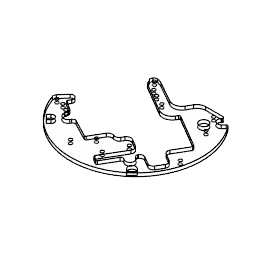
ElectronicsPlate_v18 (Autodesk Fusion 360 design; units mm, degrees)
Autodesk Fusion 360 part; units mm, degrees
sketch "Sketch1" plane through (0, 0, 0) normal (0, 0, 1) x (1, 0, 0)
  line L0 (24.0462, -23.2611) -> (4.7349, -11.9168)
  line L1 (4.7349, -11.9168) -> (-10, -37)
  line L2 (-37, -23) -> (-46.9743, -17.1407)
  line L3 (-46.9743, -17.1407) -> (-43.6068, -11.1794)
  line L4 (-43.6068, -11.1794) -> (-48.5198, -8.4041)
  circle A0 centre (0, 0) radius 60.0314
  line L5 (-48.5198, -8.4041) -> (-57.1777, -18.2887)
  line L6 (24.0462, -23.2611) -> (9.3113, -48.3442)
  line L7 (9.3113, -48.3442) -> (14.5577, -51.4261)
  line L8 (14.5577, -51.4261) -> (30.7123, -23.9261)
  line L9 (30.7123, -23.9261) -> (43.6758, -31.5414)
  line L10 (43.6758, -31.5414) -> (50.8465, -19.3347)
  line L11 (50.8465, -19.3347) -> (38.1044, -11.8495)
  line L12 (38.1044, -11.8495) -> (48.0926, 5.1535)
  line L13 (48.0926, 5.1535) -> (17.0156, 23.4093)
  line L14 (17.0156, 23.4093) -> (11.0792, 13.3037)
  line L15 (11.0792, 13.3037) -> (-19.6069, 31.3299)
  line L16 (-19.6069, 31.3299) -> (-23.3154, 25.0171)
  line L17 (-23.3154, 25.0171) -> (-29.9322, 28.904)
  line L18 (-29.9322, 28.904) -> (-25, 42)
  line L19 (-25, 42) -> (-19, 42)
  line L20 (-19, 42) -> (42.8925, 42)
  line L21 (10.662, -15.3987) -> (5.2376, -24.6327)
  line L22 (5.2376, -24.6327) -> (-0.6896, -21.1508)
  line L23 (-10, -37) -> (-37, -23)
  circle A1 centre (-45.771, -21.2236) radius 1.5
  circle A2 centre (-39.7105, -24.6734) radius 1.5
  circle A3 centre (-15.397, 31.6594) radius 1.5
  circle A4 centre (-9.3343, 28.1196) radius 1.5
  circle A5 centre (-21.7816, 38.5791) radius 1.5
  circle A6 centre (33.5, 37.5) radius 1.5
  circle A7 centre (10, -41) radius 1.5
  circle A8 centre (-3.1602, -33.1428) radius 1.5
  circle A9 centre (17.5729, -23.737) radius 1.5
  line L24 (-20.4528, 42) -> (8, 26)
  line L25 (8, 26) -> (16.9974, 42)
  circle A10 centre (-14, -46) radius 1.5
  circle A11 centre (-52.5, -20) radius 1.5
  circle A12 centre (52.7114, -12.238) radius 1.5
  circle A13 centre (41, 23) radius 1.5
  circle A14 centre (34, 28) radius 4
  circle A15 centre (28.5889, -34.0006) radius 4
  circle A16 centre (-33.8774, -28.5072) radius 4
  circle A17 centre (-27.9023, 34.2937) radius 4
  circle A18 centre (-0.4273, 23.9816) radius 1.5
  line L26 (-30.3297, -30.3548) -> (-28.4208, -27.4485)
  line L27 (-37.7611, -27.5497) -> (-37, -23)
  line L28 (-19.6069, 31.3299) -> (-23.9252, 33.8667)
  dimension "d1" = 3
  dimension "d2" = 3
  dimension "d3" = 3
  dimension "d4" = 3
  dimension "d5" = 3
  dimension "d6" = 3
  dimension "d9" = 3
  dimension "d10" = 3
  dimension "d15" = 3
  dimension "d38" = 3
  dimension "d39" = 3
  dimension "d41" = 3
  dimension "d42" = 3
  dimension "d43" = 8
  dimension "d44" = 8
  dimension "d45" = 8
  dimension "d46" = 8
  dimension "d47" = 3
  constraint perpendicular L0 L1
  constraint perpendicular L1 L2
  constraint perpendicular L3 L4
  constraint coincident A0.centre origin
  constraint coincident A0 L5.end
  constraint perpendicular L0 L6
  constraint perpendicular L6 L7
  constraint perpendicular L7 L8
  constraint perpendicular L8 L9
  constraint perpendicular L9 L10
  constraint perpendicular L8 L11
  constraint perpendicular L11 L12
  constraint perpendicular L12 L13
  constraint perpendicular L13 L14
  constraint perpendicular L14 L15
  constraint perpendicular L15 L16
  constraint perpendicular L16 L17
  constraint horizontal L19
  constraint coincident A0 L20.end
  constraint parallel L19 L20
  constraint coincident L0 L21.start
  constraint perpendicular L0 L21
  constraint coincident L1 L22.end
  constraint perpendicular L1 L22
  constraint coincident L20 L24.start
  constraint coincident L20 L25.end
  constraint perpendicular L24 L25
  constraint coincident L18 A17.centre
  constraint coincident A16 L26.start
  constraint coincident L23 L26.end
  constraint coincident A16 L27.start
  constraint coincident A17 L28.end
  constraint perpendicular L16 L28
  measures "d1" diameter of A1
  measures "d2" diameter of A2
  measures "d3" diameter of A3
  measures "d4" diameter of A4
  measures "d5" diameter of A5
  measures "d6" diameter of A6
  measures "d9" diameter of A7
  measures "d10" diameter of A8
  measures "d15" diameter of A9
  measures "d38" diameter of A10
  measures "d39" diameter of A11
  measures "d41" diameter of A12
  measures "d42" diameter of A13
  measures "d43" diameter of A14
  measures "d44" diameter of A15
  measures "d45" diameter of A16
  measures "d46" diameter of A17
  measures "d47" diameter of A18
extrude "Extrude1" add sketch "Sketch1" along normal blind 3 contours L0 L1 L2 L3 L4 A0 L5 L6 L7 L8 L9 L10 L11 L12 L13 L14 L15 L18 L19 L20 L21 L22 L23 L24 L25 A15 A16 A17 L26 L27 L28
fillet "Fillet1" radius 4 4 edges at (24.0462, -23.2611, 1.5) (10.662, -15.3987, 1.5) (5.2376, -24.6327, 1.5) (-0.6896, -21.1508, 1.5)
fillet "Fillet2" radius 1 3 edges at (14.5577, -51.4261, 1.5) (9.3113, -48.3442, 1.5) (-10, -37, 1.5)
fillet "Fillet3" radius 1 1 edges at (-46.9743, -17.1407, 1.5)
fillet "Fillet4" radius 3 3 edges at (-57.1777, -18.2887, 1.5) (-48.5198, -8.4041, 1.5) (-43.6068, -11.1794, 1.5)
fillet "Fillet5" radius 3.5 4 edges at (43.6758, -31.5414, 1.5) (30.7123, -23.9261, 1.5) (38.1044, -11.8495, 1.5) (50.8465, -19.3347, 1.5)
fillet "Fillet6" radius 1 2 edges at (48.0926, 5.1535, 1.5) (17.0156, 23.4093, 1.5)
fillet "Fillet7" radius 4 2 edges at (42.8925, 42, 1.5) (-25, 42, 1.5)
fillet "Fillet8" radius 8.5 1 edges at (11.0792, 13.3037, 1.5)
fillet "Fillet9" radius 8 2 edges at (16.9974, 42, 1.5) (8, 26, 1.5)
fillet "Fillet10" radius 14.5 1 edges at (-20.4528, 42, 1.5)
fillet "Fillet11" radius 2.5 2 edges at (-28.4208, -27.4485, 1.5) (-37, -23, 1.5)
fillet "Fillet12" radius 2 2 edges at (24.6023, -34.3272, 1.5) (26.9331, -30.3594, 1.5)
fillet "Fillet13" radius 2.5 2 edges at (-23.9252, 33.8667, 1.5) (-26.4925, 38.037, 1.5)
sketch "Sketch4" plane through (0, 0, 3) normal (0, 0, 1) x (-1, 0, 0)
  arc A0 (25.2969, -40.5706) -> (25.1203, -37.1677) centre (23.3814, -38.964) ccw
  arc A1 (23.9538, -34.9334) -> (25.1203, -37.1677) centre (27.9023, -34.2937) ccw
  arc A2 (23.9538, -34.9334) -> (22.7523, -33.1776) centre (21.486, -35.3332) ccw
  line L0 (22.7523, -33.1776) -> (-3.7502, -17.609)
  arc A3 (-3.7502, -17.609) -> (-15.3845, -20.6327) centre (-8.0555, -24.938) ccw
  line L1 (-15.3845, -20.6327) -> (-16.5091, -22.5471)
  arc A4 (-17.8778, -22.9028) -> (-16.5091, -22.5471) centre (-17.3713, -22.0406) ccw
  line L2 (-17.8778, -22.9028) -> (-47.2303, -5.66)
  arc A5 (-47.5861, -4.2912) -> (-47.2303, -5.66) centre (-46.7238, -4.7977) ccw
  line L3 (-47.5861, -4.2912) -> (-39.8772, 8.8317)
  arc A6 (-39.8772, 8.8317) -> (-41.1222, 13.6223) centre (-42.895, 10.6044) ccw
  line L4 (-41.1222, 13.6223) -> (-47.8287, 17.5619)
  arc A7 (-49.0737, 22.3525) -> (-47.8287, 17.5619) centre (-46.0559, 20.5797) ccw
  line L5 (-49.0737, 22.3525) -> (-45.4486, 28.5236)
  arc A8 (-40.658, 29.7686) -> (-45.4486, 28.5236) centre (-42.4307, 26.7508) ccw
  line L6 (-40.658, 29.7686) -> (-33.7301, 25.6989)
  arc A9 (-33.7301, 25.6989) -> (-28.9395, 26.9439) centre (-31.9573, 28.7167) ccw
  line L7 (-28.9395, 26.9439) -> (-28.7377, 27.2875)
  arc A10 (-28.7377, 27.2875) -> (-29.8377, 30.2005) centre (-30.4621, 28.3005) ccw
  arc A11 (-25.8777, 36.9416) -> (-29.8377, 30.2005) centre (-28.5889, 34.0006) ccw
  arc A12 (-25.8777, 36.9416) -> (-22.7977, 37.3991) centre (-24.5222, 38.4121) ccw
  line L8 (-22.7977, 37.3991) -> (-15.0642, 50.5639)
  arc A13 (-13.6954, 50.9196) -> (-15.0642, 50.5639) centre (-14.2019, 50.0574) ccw
  line L9 (-13.6954, 50.9196) -> (-10.1735, 48.8507)
  arc A14 (-9.8178, 47.482) -> (-10.1735, 48.8507) centre (-10.6801, 47.9885) ccw
  line L10 (-9.8178, 47.482) -> (-22.0201, 26.71)
  arc A15 (-22.0201, 26.71) -> (-20.5972, 21.235) centre (-18.5712, 24.6839) ccw
  line L11 (-20.5972, 21.235) -> (-14.1109, 17.4247)
  arc A16 (-14.1109, 17.4247) -> (-8.636, 18.8476) centre (-12.0849, 20.8736) ccw
  line L12 (-8.636, 18.8476) -> (-7.2636, 21.1837)
  arc A17 (-2.2942, 22.8574) -> (-7.2636, 21.1837) centre (-3.8147, 19.1577) ccw
  arc A18 (-2.2942, 22.8574) -> (2.6753, 24.5311) centre (-0.7737, 26.5572) ccw
  line L13 (2.6753, 24.5311) -> (9.5195, 36.1821)
  arc A19 (10.8421, 36.5634) -> (9.5195, 36.1821) centre (10.3818, 35.6756) ccw
  line L14 (10.8421, 36.5634) -> (26.4186, 28.4867)
  arc A20 (26.4186, 28.4867) -> (29.659, 29.3336) centre (27.5694, 30.706) ccw
  line L15 (29.659, 29.3336) -> (30.3297, 30.3548)
  arc A21 (37.7611, 27.5497) -> (30.3297, 30.3548) centre (33.8774, 28.5072) ccw
  line L16 (37.7611, 27.5497) -> (37.2839, 24.6967)
  arc A22 (37.2839, 24.6967) -> (38.4833, 22.1286) centre (39.7496, 24.2842) ccw
  line L17 (38.4833, 22.1286) -> (46.1265, 17.6387)
  arc A23 (46.4907, 16.2846) -> (46.1265, 17.6387) centre (45.62, 16.7765) ccw
  line L18 (46.4907, 16.2846) -> (45.0823, 13.7915)
  arc A24 (45.0823, 13.7915) -> (46.2188, 9.7039) centre (47.6944, 12.3159) ccw
  line L19 (46.2188, 9.7039) -> (46.3953, 9.6042)
  arc A25 (46.3953, 9.6042) -> (50.1275, 10.2396) centre (47.8708, 12.2163) ccw
  line L20 (50.1275, 10.2396) -> (56.0414, 16.9914)
  arc A26 (56.0414, 16.9914) -> (56.6139, 19.9658) centre (53.7847, 18.968) ccw
  arc A27 (56.6139, 19.9658) -> (-44.1162, -40.7128) centre (0, 0) ccw
  arc A28 (-44.1162, -40.7128) -> (-41.1766, -42) centre (-41.1766, -38) ccw
  line L21 (-41.1766, -42) -> (-21.6768, -42)
  arc A29 (-21.6768, -42) -> (-14.7037, -37.9212) centre (-21.6768, -34) ccw
  line L22 (-14.7037, -37.9212) -> (-11.9212, -32.9731)
  arc A30 (-1.0269, -29.9212) -> (-11.9212, -32.9731) centre (-4.9481, -36.8943) ccw
  line L23 (-1.0269, -29.9212) -> (17.4875, -40.3325)
  arc A31 (17.4875, -40.3325) -> (22.2322, -42) centre (24.5947, -27.6938) ccw
  arc A32 (22.2322, -42) -> (25.2969, -40.5706) centre (22.2322, -38) ccw
  circle A33 centre (45.771, 21.2236) radius 1.5
  circle A34 centre (39.7105, 24.6734) radius 1.5
  circle A35 centre (15.397, -31.6594) radius 1.5
  circle A36 centre (9.3343, -28.1196) radius 1.5
  circle A37 centre (21.7816, -38.5791) radius 1.5
  circle A38 centre (-33.5, -37.5) radius 1.5
  circle A39 centre (-10, 41) radius 1.5
  circle A40 centre (3.1602, 33.1428) radius 1.5
  circle A41 centre (-17.5729, 23.737) radius 1.5
  circle A42 centre (14, 46) radius 1.5
  circle A43 centre (52.5, 20) radius 1.5
  circle A44 centre (-52.7114, 12.238) radius 1.5
  circle A45 centre (-41, -23) radius 1.5
  circle A46 centre (-34, -28) radius 4
  circle A47 centre (0.4273, -23.9816) radius 1.5
sketch "Sketch5" plane through (0, 0, 0) normal (0, 0, -1) x (1, 0, 0)
  circle A0 centre (-0.4273, -23.9816) radius 1.5
  circle A1 centre (34, -28) radius 4
  circle A2 centre (41, -23) radius 1.5
  circle A3 centre (52.7114, 12.238) radius 1.5
  circle A4 centre (-52.5, 20) radius 1.5
  circle A5 centre (-14, 46) radius 1.5
  circle A6 centre (17.5729, 23.737) radius 1.5
  circle A7 centre (-3.1602, 33.1428) radius 1.5
  circle A8 centre (10, 41) radius 1.5
  circle A9 centre (33.5, -37.5) radius 1.5
  circle A10 centre (-21.7816, -38.5791) radius 1.5
  circle A11 centre (-9.3343, -28.1196) radius 1.5
  circle A12 centre (-15.397, -31.6594) radius 1.5
  circle A13 centre (-39.7105, 24.6734) radius 1.5
  circle A14 centre (-45.771, 21.2236) radius 1.5
  arc A15 (-25.1203, -37.1677) -> (-25.2969, -40.5706) centre (-23.3814, -38.964) ccw
  arc A16 (-25.2969, -40.5706) -> (-22.2322, -42) centre (-22.2322, -38) ccw
  arc A17 (-22.2322, -42) -> (-17.4875, -40.3325) centre (-24.5947, -27.6938) ccw
  line L0 (-17.4875, -40.3325) -> (1.0269, -29.9212)
  arc A18 (11.9212, -32.9731) -> (1.0269, -29.9212) centre (4.9481, -36.8943) ccw
  line L1 (11.9212, -32.9731) -> (14.7037, -37.9212)
  arc A19 (14.7037, -37.9212) -> (21.6768, -42) centre (21.6768, -34) ccw
  line L2 (21.6768, -42) -> (41.1766, -42)
  arc A20 (41.1766, -42) -> (44.1162, -40.7128) centre (41.1766, -38) ccw
  arc A21 (44.1162, -40.7128) -> (-56.6139, 19.9658) centre (0, 0) ccw
  arc A22 (-56.6139, 19.9658) -> (-56.0414, 16.9914) centre (-53.7847, 18.968) ccw
  line L3 (-56.0414, 16.9914) -> (-50.1275, 10.2396)
  arc A23 (-50.1275, 10.2396) -> (-46.3953, 9.6042) centre (-47.8708, 12.2163) ccw
  line L4 (-46.3953, 9.6042) -> (-46.2188, 9.7039)
  arc A24 (-46.2188, 9.7039) -> (-45.0823, 13.7915) centre (-47.6944, 12.3159) ccw
  line L5 (-45.0823, 13.7915) -> (-46.4907, 16.2846)
  arc A25 (-46.1265, 17.6387) -> (-46.4907, 16.2846) centre (-45.62, 16.7765) ccw
  line L6 (-46.1265, 17.6387) -> (-38.4833, 22.1286)
  arc A26 (-38.4833, 22.1286) -> (-37.2839, 24.6967) centre (-39.7496, 24.2842) ccw
  line L7 (-37.2839, 24.6967) -> (-37.7611, 27.5497)
  arc A27 (-30.3297, 30.3548) -> (-37.7611, 27.5497) centre (-33.8774, 28.5072) ccw
  line L8 (-30.3297, 30.3548) -> (-29.659, 29.3336)
  arc A28 (-29.659, 29.3336) -> (-26.4186, 28.4867) centre (-27.5694, 30.706) ccw
  line L9 (-26.4186, 28.4867) -> (-10.8421, 36.5634)
  arc A29 (-9.5195, 36.1821) -> (-10.8421, 36.5634) centre (-10.3818, 35.6756) ccw
  line L10 (-9.5195, 36.1821) -> (-2.6753, 24.5311)
  arc A30 (-2.6753, 24.5311) -> (2.2942, 22.8574) centre (0.7737, 26.5572) ccw
  arc A31 (7.2636, 21.1837) -> (2.2942, 22.8574) centre (3.8147, 19.1577) ccw
  line L11 (7.2636, 21.1837) -> (8.636, 18.8476)
  arc A32 (8.636, 18.8476) -> (14.1109, 17.4247) centre (12.0849, 20.8736) ccw
  line L12 (14.1109, 17.4247) -> (20.5972, 21.235)
  arc A33 (20.5972, 21.235) -> (22.0201, 26.71) centre (18.5712, 24.6839) ccw
  line L13 (22.0201, 26.71) -> (9.8178, 47.482)
  arc A34 (10.1735, 48.8507) -> (9.8178, 47.482) centre (10.6801, 47.9885) ccw
  line L14 (10.1735, 48.8507) -> (13.6954, 50.9196)
  arc A35 (15.0642, 50.5639) -> (13.6954, 50.9196) centre (14.2019, 50.0574) ccw
  line L15 (15.0642, 50.5639) -> (22.7977, 37.3991)
  arc A36 (22.7977, 37.3991) -> (25.8777, 36.9416) centre (24.5222, 38.4121) ccw
  arc A37 (29.8377, 30.2005) -> (25.8777, 36.9416) centre (28.5889, 34.0006) ccw
  arc A38 (29.8377, 30.2005) -> (28.7377, 27.2875) centre (30.4621, 28.3005) ccw
  line L16 (28.7377, 27.2875) -> (28.9395, 26.9439)
  arc A39 (28.9395, 26.9439) -> (33.7301, 25.6989) centre (31.9573, 28.7167) ccw
  line L17 (33.7301, 25.6989) -> (40.658, 29.7686)
  arc A40 (45.4486, 28.5236) -> (40.658, 29.7686) centre (42.4307, 26.7508) ccw
  line L18 (45.4486, 28.5236) -> (49.0737, 22.3525)
  arc A41 (47.8287, 17.5619) -> (49.0737, 22.3525) centre (46.0559, 20.5797) ccw
  line L19 (47.8287, 17.5619) -> (41.1222, 13.6223)
  arc A42 (41.1222, 13.6223) -> (39.8772, 8.8317) centre (42.895, 10.6044) ccw
  line L20 (39.8772, 8.8317) -> (47.5861, -4.2912)
  arc A43 (47.2303, -5.66) -> (47.5861, -4.2912) centre (46.7238, -4.7977) ccw
  line L21 (47.2303, -5.66) -> (17.8778, -22.9028)
  arc A44 (16.5091, -22.5471) -> (17.8778, -22.9028) centre (17.3713, -22.0406) ccw
  line L22 (16.5091, -22.5471) -> (15.3845, -20.6327)
  arc A45 (15.3845, -20.6327) -> (3.7502, -17.609) centre (8.0555, -24.938) ccw
  line L23 (3.7502, -17.609) -> (-22.7523, -33.1776)
  arc A46 (-22.7523, -33.1776) -> (-23.9538, -34.9334) centre (-21.486, -35.3332) ccw
  arc A47 (-25.1203, -37.1677) -> (-23.9538, -34.9334) centre (-27.9023, -34.2937) ccw
  circle A48 centre (-40.8476, 37.0846) radius 3
  line L24 (-40.8491, 41.3272) -> (-45.0903, 37.0831)
  line L25 (-40.8491, 41.3272) -> (-38.727, 39.2066)
  line L26 (-45.0903, 37.0831) -> (-42.9683, 34.9625)
  line L27 (-37.0831, -45.0903) -> (-34.9625, -42.9683)
  circle A49 centre (-37.0846, -40.8476) radius 3
  line L28 (-41.3272, -40.8491) -> (-37.0831, -45.0903)
  line L29 (-41.3272, -40.8491) -> (-39.2066, -38.727)
  line L30 (45.0903, -37.0831) -> (42.9683, -34.9625)
  circle A50 centre (40.8476, -37.0846) radius 3
  line L31 (40.8491, -41.3272) -> (45.0903, -37.0831)
  line L32 (40.8491, -41.3272) -> (38.727, -39.2066)
  line L33 (37.0831, 45.0903) -> (34.9625, 42.9683)
  circle A51 centre (37.0846, 40.8476) radius 3
  line L34 (41.3272, 40.8491) -> (37.0831, 45.0903)
  line L35 (41.3272, 40.8491) -> (39.2066, 38.727)
  point P0 (-42.9697, 39.2052)
  dimension "d54" = 6
  dimension "d55" = 6
  dimension "d57" = 360
  constraint midpoint L24 P0
  constraint coincident A48 P0
  constraint coincident A48 L25.end
  constraint tangent A48 L25
  constraint coincident A48 L26.end
  constraint perpendicular L24 L26
  constraint tangent A48 L26
  measures "d54" diameter of A48
  measures "d55" distance of L24.start L24.end
extrude "Extrude2" cut sketch "Sketch5" against normal blind 7 contours A48 | A48 L24 L25 | A48 L24 L26 | L30 A50 L31 | A50 | A50 L31 L32 | L33 A51 L34 | A51 | A51 L34 L35
sketch "Sketch6" plane through (0, 0, 0) normal (0, 0, -1) x (1, 0, 0)
  circle A0 centre (41, -23) radius 1.5
  circle A1 centre (-9.3343, -28.1196) radius 1.5
  circle A2 centre (-14, 46) radius 1.5
  circle A3 centre (34, -28) radius 4
  circle A4 centre (17.5729, 23.737) radius 1.5
  circle A5 centre (33.5, -37.5) radius 1.5
  circle A6 centre (-39.7105, 24.6734) radius 1.5
  circle A7 centre (-15.397, -31.6594) radius 1.5
  circle A8 centre (-3.1602, 33.1428) radius 1.5
  circle A9 centre (-45.771, 21.2236) radius 1.5
  circle A10 centre (52.7114, 12.238) radius 1.5
  circle A11 centre (-52.5, 20) radius 1.5
  circle A12 centre (10, 41) radius 1.5
  circle A13 centre (-0.4273, -23.9816) radius 1.5
  circle A14 centre (-21.7816, -38.5791) radius 1.5
  arc A15 (-25.1203, -37.1677) -> (-25.2969, -40.5706) centre (-23.3814, -38.964) ccw
  arc A16 (-25.2969, -40.5706) -> (-22.2322, -42) centre (-22.2322, -38) ccw
  arc A17 (-22.2322, -42) -> (-17.4875, -40.3325) centre (-24.5947, -27.6938) ccw
  line L0 (-17.4875, -40.3325) -> (1.0269, -29.9212)
  arc A18 (11.9212, -32.9731) -> (1.0269, -29.9212) centre (4.9481, -36.8943) ccw
  line L1 (11.9212, -32.9731) -> (14.7037, -37.9212)
  arc A19 (14.7037, -37.9212) -> (21.6768, -42) centre (21.6768, -34) ccw
  line L2 (21.6768, -42) -> (41.1766, -42)
  arc A20 (41.1766, -42) -> (44.1162, -40.7128) centre (41.1766, -38) ccw
  arc A21 (44.1162, -40.7128) -> (-56.6139, 19.9658) centre (0, 0) ccw
  arc A22 (-56.6139, 19.9658) -> (-56.0414, 16.9914) centre (-53.7847, 18.968) ccw
  line L3 (-56.0414, 16.9914) -> (-50.1275, 10.2396)
  arc A23 (-50.1275, 10.2396) -> (-46.3953, 9.6042) centre (-47.8708, 12.2163) ccw
  line L4 (-46.3953, 9.6042) -> (-46.2188, 9.7039)
  arc A24 (-46.2188, 9.7039) -> (-45.0823, 13.7915) centre (-47.6944, 12.3159) ccw
  line L5 (-45.0823, 13.7915) -> (-46.4907, 16.2846)
  arc A25 (-46.1265, 17.6387) -> (-46.4907, 16.2846) centre (-45.62, 16.7765) ccw
  line L6 (-46.1265, 17.6387) -> (-38.4833, 22.1286)
  arc A26 (-38.4833, 22.1286) -> (-37.2839, 24.6967) centre (-39.7496, 24.2842) ccw
  line L7 (-37.2839, 24.6967) -> (-37.7611, 27.5497)
  arc A27 (-30.3297, 30.3548) -> (-37.7611, 27.5497) centre (-33.8774, 28.5072) ccw
  line L8 (-30.3297, 30.3548) -> (-29.659, 29.3336)
  arc A28 (-29.659, 29.3336) -> (-26.4186, 28.4867) centre (-27.5694, 30.706) ccw
  line L9 (-26.4186, 28.4867) -> (-10.8421, 36.5634)
  arc A29 (-9.5195, 36.1821) -> (-10.8421, 36.5634) centre (-10.3818, 35.6756) ccw
  line L10 (-9.5195, 36.1821) -> (-2.6753, 24.5311)
  arc A30 (-2.6753, 24.5311) -> (2.2942, 22.8574) centre (0.7737, 26.5572) ccw
  arc A31 (7.2636, 21.1837) -> (2.2942, 22.8574) centre (3.8147, 19.1577) ccw
  line L11 (7.2636, 21.1837) -> (8.636, 18.8476)
  arc A32 (8.636, 18.8476) -> (14.1109, 17.4247) centre (12.0849, 20.8736) ccw
  line L12 (14.1109, 17.4247) -> (20.5972, 21.235)
  arc A33 (20.5972, 21.235) -> (22.0201, 26.71) centre (18.5712, 24.6839) ccw
  line L13 (22.0201, 26.71) -> (9.8178, 47.482)
  arc A34 (10.1735, 48.8507) -> (9.8178, 47.482) centre (10.6801, 47.9885) ccw
  line L14 (10.1735, 48.8507) -> (13.6954, 50.9196)
  arc A35 (15.0642, 50.5639) -> (13.6954, 50.9196) centre (14.2019, 50.0574) ccw
  line L15 (15.0642, 50.5639) -> (22.7977, 37.3991)
  arc A36 (22.7977, 37.3991) -> (25.8777, 36.9416) centre (24.5222, 38.4121) ccw
  arc A37 (29.8377, 30.2005) -> (25.8777, 36.9416) centre (28.5889, 34.0006) ccw
  arc A38 (29.8377, 30.2005) -> (28.7377, 27.2875) centre (30.4621, 28.3005) ccw
  line L16 (28.7377, 27.2875) -> (28.9395, 26.9439)
  arc A39 (28.9395, 26.9439) -> (33.7301, 25.6989) centre (31.9573, 28.7167) ccw
  line L17 (33.7301, 25.6989) -> (40.658, 29.7686)
  arc A40 (45.4486, 28.5236) -> (40.658, 29.7686) centre (42.4307, 26.7508) ccw
  line L18 (45.4486, 28.5236) -> (49.0737, 22.3525)
  arc A41 (47.8287, 17.5619) -> (49.0737, 22.3525) centre (46.0559, 20.5797) ccw
  line L19 (47.8287, 17.5619) -> (41.1222, 13.6223)
  arc A42 (41.1222, 13.6223) -> (39.8772, 8.8317) centre (42.895, 10.6044) ccw
  line L20 (39.8772, 8.8317) -> (47.5861, -4.2912)
  arc A43 (47.2303, -5.66) -> (47.5861, -4.2912) centre (46.7238, -4.7977) ccw
  line L21 (47.2303, -5.66) -> (17.8778, -22.9028)
  arc A44 (16.5091, -22.5471) -> (17.8778, -22.9028) centre (17.3713, -22.0406) ccw
  line L22 (16.5091, -22.5471) -> (15.3845, -20.6327)
  arc A45 (15.3845, -20.6327) -> (3.7502, -17.609) centre (8.0555, -24.938) ccw
  line L23 (3.7502, -17.609) -> (-22.7523, -33.1776)
  arc A46 (-22.7523, -33.1776) -> (-23.9538, -34.9334) centre (-21.486, -35.3332) ccw
  arc A47 (-25.1203, -37.1677) -> (-23.9538, -34.9334) centre (-27.9023, -34.2937) ccw
  line L24 (42.9683, -34.9625) -> (45.0903, -37.0831)
  line L25 (45.0903, -37.0831) -> (40.8491, -41.3272)
  line L26 (40.8491, -41.3272) -> (38.727, -39.2066)
  arc A48 (42.9683, -34.9625) -> (38.727, -39.2066) centre (40.8476, -37.0846) ccw
  line L27 (37.0831, 45.0903) -> (41.3272, 40.8491)
  line L28 (41.3272, 40.8491) -> (39.2066, 38.727)
  arc A49 (34.9625, 42.9683) -> (39.2066, 38.727) centre (37.0846, 40.8476) ccw
  line L29 (34.9625, 42.9683) -> (37.0831, 45.0903)
  line L30 (-42.9683, 34.9625) -> (-45.0903, 37.0831)
  line L31 (-45.0903, 37.0831) -> (-40.8491, 41.3272)
  line L32 (-40.8491, 41.3272) -> (-38.727, 39.2066)
  arc A50 (-42.9683, 34.9625) -> (-38.727, 39.2066) centre (-40.8476, 37.0846) ccw
  line L33 (-40.8488, 40.6201) -> (-39.0805, 38.8529)
  arc A51 (-42.6148, 35.3162) -> (-39.0805, 38.8529) centre (-40.8476, 37.0846) ccw
  line L34 (-42.6148, 35.3162) -> (-44.3832, 37.0834)
  line L35 (-44.3832, 37.0834) -> (-40.8488, 40.6201)
  line L36 (42.0343, 40.8493) -> (39.5603, 38.3736)
  arc A52 (34.6089, 43.3217) -> (39.5603, 38.3736) centre (37.0846, 40.8476) ccw
  line L37 (34.6089, 43.3217) -> (37.0829, 45.7974)
  line L38 (37.0829, 45.7974) -> (42.0343, 40.8493)
  arc A53 (43.3217, -34.6089) -> (38.3736, -39.5603) centre (40.8476, -37.0846) ccw
  line L39 (40.8493, -42.0343) -> (38.3736, -39.5603)
  line L40 (45.7974, -37.0829) -> (40.8493, -42.0343)
  line L41 (43.3217, -34.6089) -> (45.7974, -37.0829)
  line L42 (45.7974, -37.0829) -> (46.5819, -37.8668)
  dimension "d60" = 0.5
  dimension "d61" = 0.5
  dimension "d62" = -0.5
  constraint coincident A21 L42.end
  constraint perpendicular L40 L42
extrude "Extrude3" cut sketch "Sketch6" against normal blind 8 contours L2 A53 L39 L40 L41 | L2 A20 A21 L40 L42 | L30 L31 L32 A50 | L36 A52 L37 L38
fillet "Fillet14" radius 1.25 2 edges at (46.5819, 37.8668, 1.5) (40.815, 42, 1.5)
sketch "Sketch7" plane through (0, 0, 3) normal (0, 0, 1) x (-1, 0, 0)
  arc A0 (-38.6794, -39.8658) -> (-37.7958, -42) centre (-37.7958, -40.75) ccw
  line L0 (-37.7958, -42) -> (-21.6768, -42)
  arc A1 (-21.6768, -42) -> (-14.7037, -37.9212) centre (-21.6768, -34) ccw
  line L1 (-14.7037, -37.9212) -> (-11.9212, -32.9731)
  arc A2 (-1.0269, -29.9212) -> (-11.9212, -32.9731) centre (-4.9481, -36.8943) ccw
  line L2 (-1.0269, -29.9212) -> (17.4875, -40.3325)
  arc A3 (17.4875, -40.3325) -> (22.2322, -42) centre (24.5947, -27.6938) ccw
  arc A4 (22.2322, -42) -> (25.2969, -40.5706) centre (22.2322, -38) ccw
  arc A5 (25.2969, -40.5706) -> (25.1203, -37.1677) centre (23.3814, -38.964) ccw
  arc A6 (23.9538, -34.9334) -> (25.1203, -37.1677) centre (27.9023, -34.2937) ccw
  arc A7 (23.9538, -34.9334) -> (22.7523, -33.1776) centre (21.486, -35.3332) ccw
  line L3 (22.7523, -33.1776) -> (-3.7502, -17.609)
  arc A8 (-3.7502, -17.609) -> (-15.3845, -20.6327) centre (-8.0555, -24.938) ccw
  line L4 (-15.3845, -20.6327) -> (-16.5091, -22.5471)
  arc A9 (-17.8778, -22.9028) -> (-16.5091, -22.5471) centre (-17.3713, -22.0406) ccw
  line L5 (-17.8778, -22.9028) -> (-47.2303, -5.66)
  arc A10 (-47.5861, -4.2912) -> (-47.2303, -5.66) centre (-46.7238, -4.7977) ccw
  line L6 (-47.5861, -4.2912) -> (-39.8772, 8.8317)
  arc A11 (-39.8772, 8.8317) -> (-41.1222, 13.6223) centre (-42.895, 10.6044) ccw
  line L7 (-41.1222, 13.6223) -> (-47.8287, 17.5619)
  arc A12 (-49.0737, 22.3525) -> (-47.8287, 17.5619) centre (-46.0559, 20.5797) ccw
  line L8 (-49.0737, 22.3525) -> (-45.4486, 28.5236)
  arc A13 (-40.658, 29.7686) -> (-45.4486, 28.5236) centre (-42.4307, 26.7508) ccw
  line L9 (-40.658, 29.7686) -> (-33.7301, 25.6989)
  arc A14 (-33.7301, 25.6989) -> (-28.9395, 26.9439) centre (-31.9573, 28.7167) ccw
  line L10 (-28.9395, 26.9439) -> (-28.7377, 27.2875)
  arc A15 (-28.7377, 27.2875) -> (-29.8377, 30.2005) centre (-30.4621, 28.3005) ccw
  arc A16 (-25.8777, 36.9416) -> (-29.8377, 30.2005) centre (-28.5889, 34.0006) ccw
  arc A17 (-25.8777, 36.9416) -> (-22.7977, 37.3991) centre (-24.5222, 38.4121) ccw
  line L11 (-22.7977, 37.3991) -> (-15.0642, 50.5639)
  arc A18 (-13.6954, 50.9196) -> (-15.0642, 50.5639) centre (-14.2019, 50.0574) ccw
  line L12 (-13.6954, 50.9196) -> (-10.1735, 48.8507)
  arc A19 (-9.8178, 47.482) -> (-10.1735, 48.8507) centre (-10.6801, 47.9885) ccw
  line L13 (-9.8178, 47.482) -> (-22.0201, 26.71)
  arc A20 (-22.0201, 26.71) -> (-20.5972, 21.235) centre (-18.5712, 24.6839) ccw
  line L14 (-20.5972, 21.235) -> (-14.1109, 17.4247)
  arc A21 (-14.1109, 17.4247) -> (-8.636, 18.8476) centre (-12.0849, 20.8736) ccw
  line L15 (-8.636, 18.8476) -> (-7.2636, 21.1837)
  arc A22 (-2.2942, 22.8574) -> (-7.2636, 21.1837) centre (-3.8147, 19.1577) ccw
  arc A23 (-2.2942, 22.8574) -> (2.6753, 24.5311) centre (-0.7737, 26.5572) ccw
  line L16 (2.6753, 24.5311) -> (9.5195, 36.1821)
  arc A24 (10.8421, 36.5634) -> (9.5195, 36.1821) centre (10.3818, 35.6756) ccw
  line L17 (10.8421, 36.5634) -> (26.4186, 28.4867)
  arc A25 (26.4186, 28.4867) -> (29.659, 29.3336) centre (27.5694, 30.706) ccw
  line L18 (29.659, 29.3336) -> (30.3297, 30.3548)
  arc A26 (37.7611, 27.5497) -> (30.3297, 30.3548) centre (33.8774, 28.5072) ccw
  line L19 (37.7611, 27.5497) -> (37.2839, 24.6967)
  arc A27 (37.2839, 24.6967) -> (38.4833, 22.1286) centre (39.7496, 24.2842) ccw
  line L20 (38.4833, 22.1286) -> (46.1265, 17.6387)
  arc A28 (46.4907, 16.2846) -> (46.1265, 17.6387) centre (45.62, 16.7765) ccw
  line L21 (46.4907, 16.2846) -> (45.0823, 13.7915)
  arc A29 (45.0823, 13.7915) -> (46.2188, 9.7039) centre (47.6944, 12.3159) ccw
  line L22 (46.2188, 9.7039) -> (46.3953, 9.6042)
  arc A30 (46.3953, 9.6042) -> (50.1275, 10.2396) centre (47.8708, 12.2163) ccw
  line L23 (50.1275, 10.2396) -> (56.0414, 16.9914)
  arc A31 (56.0414, 16.9914) -> (56.6139, 19.9658) centre (53.7847, 18.968) ccw
  arc A32 (56.6139, 19.9658) -> (-47.4623, -36.7573) centre (0, 0) ccw
  arc A33 (-47.4623, -36.7573) -> (-45.5904, -36.8761) centre (-46.474, -35.9919) ccw
  line L24 (-45.5904, -36.8761) -> (-43.3217, -34.6089)
  arc A34 (-38.3736, -39.5603) -> (-43.3217, -34.6089) centre (-40.8476, -37.0846) ccw
  line L25 (-38.3736, -39.5603) -> (-38.6794, -39.8658)
  line L26 (45.0903, 37.0831) -> (42.9683, 34.9625)
  arc A35 (38.727, 39.2066) -> (42.9683, 34.9625) centre (40.8476, 37.0846) ccw
  line L27 (38.727, 39.2066) -> (40.8491, 41.3272)
  line L28 (40.8491, 41.3272) -> (45.0903, 37.0831)
  circle A36 centre (-41, -23) radius 1.5
  circle A37 centre (9.3343, -28.1196) radius 1.5
  circle A38 centre (14, 46) radius 1.5
  circle A39 centre (-34, -28) radius 4
  circle A40 centre (-17.5729, 23.737) radius 1.5
  circle A41 centre (-33.5, -37.5) radius 1.5
  circle A42 centre (39.7105, 24.6734) radius 1.5
  circle A43 centre (15.397, -31.6594) radius 1.5
  circle A44 centre (3.1602, 33.1428) radius 1.5
  circle A45 centre (45.771, 21.2236) radius 1.5
  circle A46 centre (-52.7114, 12.238) radius 1.5
  circle A47 centre (52.5, 20) radius 1.5
  circle A48 centre (-10, 41) radius 1.5
  circle A49 centre (0.4273, -23.9816) radius 1.5
  circle A50 centre (21.7816, -38.5791) radius 1.5
  line L29 (-39.5603, 38.3736) -> (-42.0343, 40.8493)
  line L30 (-42.0343, 40.8493) -> (-37.0829, 45.7974)
  line L31 (-37.0829, 45.7974) -> (-34.6089, 43.3217)
  arc A51 (-39.5603, 38.3736) -> (-34.6089, 43.3217) centre (-37.0846, 40.8476) ccw
